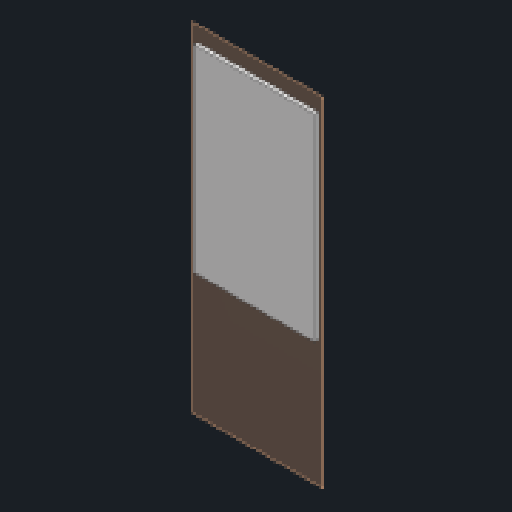
# Autodesk Inventor part: right_metal_gear_bracker
Saved by Autodesk Inventor 2023 (Build 270158000, 158)
## iProperties
Created: 2024-04-23
Part Number: right_metal_gear_bracker
Material: Generic
Document SubType Name: Modeling
Designer: szymo
Density: 1 g/cm^3
Appearance: Default
Author: szymo
Autodesk Inventor part; units mm, degrees
ref_plane "YZ Plane" through (0, 0, 0) normal (1, 0, 0) x (0, 1, 0)
ref_plane "XZ Plane" through (0, 0, 0) normal (0, 1, 0) x (-1, 0, 0)
ref_plane "XY Plane" through (0, 0, 0) normal (0, 0, 1) x (1, 0, 0)
ref_plane "Work Plane1" through (3, 0, -1) normal (0, 0, 1) x (0, -1, 0)
sketch "Sketch1" plane through (3, 0, -1) normal (0, 0, 1) x (0, -1, 0)
  line L0 (85.75, 33.5) -> (0, 33.5) projected
  line L1 (0, 0) -> (0, 33.5) projected
  line L2 (0, 0) -> (85.75, 0) projected
  line L3 (85.75, 0) -> (85.75, 33.5) projected
  line L4 (52, 0) -> (52, -3) projected
  line L5 (0, 0) -> (52, 0) projected
  line L6 (0, -3) -> (0, 0) projected
  line L7 (0, -3) -> (52, -3) projected
  line L8 (55, 0) -> (175, 0) projected
  line L9 (175, 0) -> (175, 4.5) projected
  line L10 (175, 4.5) -> (129.8889, 33.5) projected
  line L11 (129.8889, 33.5) -> (55, 33.5) projected
  line L12 (55, 33.5) -> (55, 0) projected
extrude "Extrusion1" add sketch "Sketch1" along normal blind 1 contours L12 L2 L1 L0
body "Solid1"
